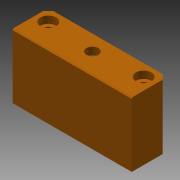
# Autodesk Inventor part: Peripherie2_Motor2_liegend
Saved by Autodesk Inventor 2015 (Build 190159000, 159)
## iProperties
Created: 2015-03-02
Part Number: Peripherie2_Motor2_liegend
Material: Generisch
Document SubType Name: Modeling
Designer: TowerSebi
Density: 1 g/cm^3
Appearance: Orange
Author: TowerSebi
Autodesk Inventor part; units mm, degrees
ref_plane "YZ Plane" through (0, 0, 0) normal (1, 0, 0) x (0, 1, 0)
ref_plane "XZ Plane" through (0, 0, 0) normal (0, 1, 0) x (-1, 0, 0)
ref_plane "XY Plane" through (0, 0, 0) normal (0, 0, 1) x (1, 0, 0)
sketch "Skizze1" plane through (0, 0, 0) normal (0, 0, 1) x (1, 0, 0)
  line L0 (0, 0) -> (50, 0)
  line L1 (50, 0) -> (50, 15)
  line L2 (50, 15) -> (0, 15)
  line L3 (0, 15) -> (0, 0)
  dimension "d0" = 15
  dimension "d1" = 50
  constraints: 8 end point, 2 parallel, 1 horizontal, 1 perpendicular
  measures "d0" distance of L2.end L0.start
  measures "d1" distance of L0.start L0.end
extrude "Extrusion1" add sketch "Skizze1" along normal blind 28.5
hole "Bohrung1" at (45, 10, 28.5) direction (0, 0, -1) diameter 3.4 end through all counterbore diameter 6.5 counterbore depth 3 clearance for "Inbusschraube DIN EN ISO 4762" size "M3" standard "DIN"
hole "Bohrung2" at (5, 10, 28.5) direction (0, 0, -1) diameter 3.4 end through all counterbore diameter 6.5 counterbore depth 3 clearance for "Inbusschraube DIN EN ISO 4762" size "M3" standard "DIN"
chamfer "Fase1" distance 0.5 angle 45 1 edges at (25, 0, 28.5)
sketch "Skizze2" plane through (0, 0, 0) normal (0, 0, -1) x (-1, 0, 0)
  line L0 (0, 15) -> (0, 0) projected
  line L1 (-50, 15) -> (0, 15) projected
  line L2 (-50, 0) -> (-50, 15) projected
  line L3 (-40, 15) -> (-10, 15)
  line L4 (-10, 15) -> (-10, 2)
  line L5 (-10, 2) -> (-40, 2)
  line L6 (-40, 2) -> (-40, 15)
  line L7 (0, 0) -> (-50, 0) projected
  dimension "d25" = 10
  dimension "d26" = 10
  dimension "d44" = 2
  constraints: 8 end point, 2 parallel, 1 horizontal, 1 perpendicular, 1 point on line
  measures "d25" distance between parallel lines of L2 L6
  measures "d26" distance between parallel lines of L0 L4
  measures "d44" distance between parallel lines of L7 L5
extrude "Extrusion2" cut sketch "Skizze2" against normal blind 25.5 contours L4 L5 L6 L1
hole "Bohrung3" at (25, 8.5, 28.5) direction (0, 0, -1) diameter 5 end through all
chamfer "Fase2" distance 2 angle 45 2 edges at (50, 15, 14.25) (0, 15, 14.25)
sketch "Skizze4" plane through (0, 0, 0) normal (0, 0, -1) x (-1, 0, 0)
  line L0 (-50, 0) -> (-50, 13)
  line L1 (-50, 0) -> (-50, 13) projected
  line L2 (-50, 13) -> (-48, 15)
  line L3 (-48, 15) -> (-50, 13) projected
  line L4 (-48, 15) -> (-40, 15)
  line L5 (-48, 15) -> (-40, 15) projected
  line L6 (-40, 15) -> (-40, 3)
  line L7 (-40, 2) -> (-40, 15) projected
  line L8 (-40, 2) -> (-10, 2)
  line L9 (-10, 2) -> (-40, 2) projected
  line L10 (-10, 2) -> (-10, 15)
  line L11 (-10, 15) -> (-10, 2) projected
  line L12 (-10, 15) -> (-2, 15)
  line L13 (-2, 15) -> (0, 13)
  line L14 (0, 13) -> (-2, 15) projected
  line L15 (0, 13) -> (0, 0)
  line L16 (0, 0) -> (-50, 0)
  line L17 (0, 0) -> (-50, 0) projected
  constraints: 20 end point, 8 equal length, 1 perpendicular, 1 point on line
extrude "Extrusion4" cut sketch "Skizze4" against normal blind 1.5
